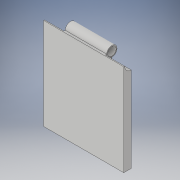
# Autodesk Inventor part: outerFrontPlate
Saved by Autodesk Inventor 2019 (Build 230136000, 136)
## iProperties
Created: 2018-07-23
Part Number: outerFrontPlate
Material: Generic
Document SubType Name: Modeling
Designer: Ge Shi
Density: 1 g/cm^3
Appearance: Default
Author: Ge Shi
Autodesk Inventor part; units mm, degrees
ref_plane "YZ Plane" through (0, 0, 0) normal (1, 0, 0) x (0, 1, 0)
ref_plane "XZ Plane" through (0, 0, 0) normal (0, 1, 0) x (-1, 0, 0)
ref_plane "XY Plane" through (0, 0, 0) normal (0, 0, 1) x (1, 0, 0)
sketch "Sketch1" plane through (0, 0, 0) normal (0, 0, 1) x (1, 0, 0)
  line L0 (21.5, -24.625) -> (-21.5, -24.625)
  line L1 (-21.5, -24.625) -> (-21.5, 24.625)
  line L2 (-21.5, 24.625) -> (21.5, 24.625)
  line L3 (21.5, 24.625) -> (21.5, -24.625)
  line L4 (21.5, -24.625) -> (-21.5, 24.625) construction
  line L5 (-21.5, -24.625) -> (21.5, 24.625) construction
  point P0 (0, 0)
  dimension "d0" = 43
  dimension "d1" = 49.25
  constraints: 12 end point, 2 midpoint, 2 parallel, 1 horizontal, 1 perpendicular
  measures "d0" distance of L1.end L2.end
  measures "d1" distance of L0.end L1.end
extrude "Extrusion1" add sketch "Sketch1" along normal blind 4
ref_plane "Work Plane1" through (0, -24.625, 0) normal (1, 0, 0) x (0, 0, -1)
sketch "Sketch2" plane through (0, -24.625, 0) normal (1, 0, 0) x (0, 0, -1)
  circle A0 centre (0, 49.25) radius 2.25
  circle A1 centre (0, 49.25) radius 2.75
  circle A2 centre (0, 49.25) radius 3.5
  point P0 (0, 24.625)
  point P1 (0, 0)
  dimension "d4" = 4.5
  dimension "d6" = 5.5
  dimension "d7" = 7
  constraints: 3 centre point, 2 coincident
  measures "d4" diameter of A0
  measures "d6" diameter of A1
  measures "d7" diameter of A2
extrude "Extrusion2" cut sketch "Sketch2" along normal mid plane 43 contours A0 | A1
extrude "Extrusion3" add sketch "Sketch2" along normal mid plane 22.25 contours A1
extrude "Extrusion4" cut sketch "Sketch2" along normal blind 25 from surface at 11.125 contours A2
extrude "Extrusion5" cut sketch "Sketch2" against normal blind 20 from surface at -11.125 contours A2
equation "\"d0\" = -hingeShaftHolder + length - clearance"
equation "\"d1\" = 0.5 * height - 0.5 * clearance"
equation "\"d2\" = thick"
equation "\"d4\" = hingeShaft + clearance"
equation "\"d6\" = hingeShaftHolder"
equation "\"d7\" = clearance + hingeShaftHolder"
equation "\"d8\" = -hingeShaftHolder + length - clearance"
equation "\"d12\" = 0.5 * length"
equation "\"d14\" = widthOuter"
equation "\"hingeShaftHolder\" = 5.5"
equation "\"length\" = 50"
equation "\"clearance\" = 1.5"
equation "\"height\" = 100"
equation "\"thick\" = 4"
equation "\"hingeShaft\" = 3"
equation "\"widthOuter\" = 20"
body "Solid1"
